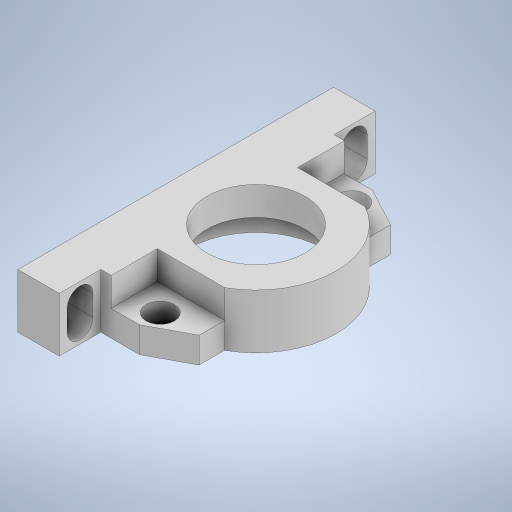
# Autodesk Inventor part: clock_part1
Saved by Autodesk Inventor 2024 (Build 280153000, 153)
## iProperties
Created: 2024-10-24
Part Number: clock_part1
Material: Generic
Document SubType Name: Modeling
Designer: Logan
Density: 1 g/cm^3
Appearance: Default
Author: Logan
Autodesk Inventor part; units mm, degrees
ref_plane "YZ Plane" through (0, 0, 0) normal (1, 0, 0) x (0, 1, 0)
ref_plane "XZ Plane" through (0, 0, 0) normal (0, 1, 0) x (-1, 0, 0)
ref_plane "XY Plane" through (0, 0, 0) normal (0, 0, 1) x (1, 0, 0)
sketch "Sketch1" plane through (0, 0, 0) normal (0, 1, 0) x (-1, 0, 0)
  circle A0 centre (0, 0) radius 13
  circle A1 centre (0, 0) radius 15.5
  circle A2 centre (0, 18.5) radius 2.75
  circle A3 centre (0, -18.5) radius 2.75
  line L0 (0, 18.5) -> (0, -18.5)
  line L1 (7.5, 22.5) -> (-7.5, 22.5)
  line L2 (-7.5, 22.5) -> (-7.5, 13)
  line L3 (-7.5, 13) -> (7.5, 13)
  line L4 (7.5, 13) -> (7.5, 22.5)
  line L5 (0, 22.5) -> (7.5, 18.5)
  line L6 (7.5, 18.5) -> (7.5, 13.5647)
  line L7 (0, 22.5) -> (-7.5, 18.5)
  line L8 (-7.5, 18.5) -> (-7.5, 13.5647)
  line L9 (13, 0) -> (-13, 0) construction
  circle A4 centre (0, -18.5) radius 2.75
  line L10 (7.5, -22.5) -> (-7.5, -22.5)
  line L11 (-7.5, -22.5) -> (-7.5, -13)
  line L12 (7.5, -13) -> (7.5, -22.5)
  line L13 (0, -22.5) -> (7.5, -18.5)
  line L14 (0, -22.5) -> (-7.5, -18.5)
  point P0 (-7.5, -13.5647)
  point P1 (7.5, -13.5647)
  dimension "d0" = 26
  dimension "d1" = 2.5
  dimension "d2" = 5.5
  dimension "d3" = 5.5
  dimension "d4" = 37
  dimension "d5" = 15
  dimension "d6" = 4
  constraints: 30 end point, 7 symmetric about line, 6 point on line, 5 centre point, 4 coincident, 4 point on circle, 2 horizontal, 2 midpoint, 2 parallel, 2 vertical alignment, 1 perpendicular, 1 tangent, 1 vertical, 1 other
  measures "d0" diameter of A0
  measures "d1" radial gap between concentric circles of A0 A1
  measures "d2" diameter of A2
  measures "d3" diameter of A3
  measures "d4" distance of L0.end L0.start
  measures "d5" distance of L3.end L2.end
  measures "d6" distance of L5.start L0.start
extrude "Extrusion1" add sketch "Sketch1" along normal blind 5 contours A0 L3 L4 A1 L0 | L3 L2 A1 L0 | A0 L0 A1 L2 L3 | L0 A1 L4 L3 | A1 L2 L7 L5 L4 | A1 L12 L13 L14 L11
sketch "Sketch2" plane through (0, 0, 0) normal (0, -1, 0) x (1, 0, 0)
  line L0 (7.5, -18.5) -> (0, -22.5) projected
  line L1 (0, -22.5) -> (-15.5, -22.5)
  line L2 (-15.5, -22.5) -> (-15.5, 22.5)
  line L3 (-15.5, 22.5) -> (0, 22.5)
  arc A0 (-7.5, 13.5647) -> (-7.5, -13.5647) centre (0, 0) ccw projected
  line L4 (-7.5, 13.5647) -> (-7.5, 18.5) projected
  line L5 (0, 22.5) -> (-7.5, 18.5)
  line L6 (-7.5, 18.5) -> (-7.5, 13.5647)
  arc A1 (-7.5, 13.5647) -> (-15.5, 0) centre (0, 0) ccw
  line L7 (0, -22.5) -> (-7.5, -18.5) projected
  line L8 (0, -22.5) -> (-7.5, -18.5)
  line L9 (-7.5, -18.5) -> (-7.5, -13.5647)
  line L10 (-7.5, -18.5) -> (-7.5, -13.5647) projected
  arc A2 (-7.5, 13.5647) -> (-7.5, -13.5647) centre (0, 0) ccw
  point P0 (-15.5, 0)
  constraints: 14 end point, 5 point on circle, 3 equal length, 2 centre point, 2 coincident, 1 concentric, 1 horizontal, 1 parallel, 1 point on line, 1 tangent, 1 vertical
extrude "Extrusion2" add sketch "Sketch2" against normal up to surface (5 mm away)
sketch "Sketch4" plane through (0, 5, 0) normal (0, 1, 0) x (1, 0, 0)
  arc A0 (7.5, -13.5647) -> (7.5, 13.5647) centre (0, 0) ccw projected
  arc A1 (7.5, -13.5647) -> (7.5, 13.5647) centre (0, 0) ccw
  line L0 (7.5, 13.5647) -> (7.5, 18.5) projected
  line L1 (7.5, 13.5647) -> (-5.5, 13.5647)
  line L2 (-5.5, 13.5647) -> (-5.5, 22.5742)
  line L3 (-5.5, 22.5742) -> (-15.5, 22.5742)
  line L4 (-15.5, -22.5) -> (-15.5, 22.5) projected
  line L5 (-15.5, 22.5742) -> (-15.5, -22.5)
  line L6 (0, -22.5) -> (-15.5, -22.5) projected
  line L7 (-15.5, -22.5) -> (-5.5, -22.5)
  line L8 (-5.5, -22.5) -> (-5.5, -13.5647)
  line L9 (-5.5, -13.5647) -> (7.5, -13.5647)
  line L10 (7.5, -18.5) -> (7.5, -13.5647) projected
  circle A2 centre (0, 0) radius 9.5
  point P0 (-15.5, -30.5)
  point P1 (-15.5, 30.5)
  point P2 (-10, -22.5)
  point P3 (-15.5, -22.5)
  point P4 (-5.5, -22.5)
  point P5 (-5.5, -22.5)
  dimension "d21" = 13
  dimension "d22" = 13
  dimension "d23" = 19
  constraints: 14 end point, 5 perpendicular, 2 centre point, 2 horizontal, 2 point on circle, 1 coincident, 1 point on line
  measures "d21" distance between parallel lines of L2 L0
  measures "d22" distance between parallel lines of L8 L10
  measures "d23" diameter of A2
extrude "Extrusion4" add sketch "Sketch4" along normal blind 5.5
sketch "Sketch5" plane through (-15.5, 0, -22.5) normal (-1, 0, 0) x (0, 0, 1)
  line L0 (45, 0) -> (45, 5) projected
  line L1 (45, 0) -> (53, 0)
  line L2 (53, 0) -> (53, 10.5)
  line L3 (53, 10.5) -> (45, 10.5)
  line L4 (45, 10.5) -> (45, 0)
  line L5 (4, 0) -> (0, 0) projected
  line L6 (0, 0) -> (-8, 0)
  line L7 (-8, 0) -> (-8, 10.5)
  line L8 (-8, 10.5) -> (0, 10.5)
  line L9 (0, 10.5) -> (0, 0)
  line L10 (-0.0742, 10.5) -> (45, 10.5) projected
  line L11 (-4, 3.25) -> (-4, 7.25) construction
  line L12 (-1.5, 3.25) -> (-1.5, 7.25)
  line L13 (-6.5, 7.25) -> (-6.5, 3.25)
  arc A0 (-6.5, 3.25) -> (-1.5, 3.25) centre (-4, 3.25) ccw
  arc A1 (-1.5, 7.25) -> (-6.5, 7.25) centre (-4, 7.25) ccw
  line L14 (49, 3.25) -> (49, 7.25) construction
  line L15 (51.5, 3.25) -> (51.5, 7.25)
  line L16 (46.5, 7.25) -> (46.5, 3.25)
  arc A2 (46.5, 3.25) -> (51.5, 3.25) centre (49, 3.25) ccw
  arc A3 (51.5, 7.25) -> (46.5, 7.25) centre (49, 7.25) ccw
  point P0 (22.5, 0)
  point P1 (49, 10.5)
  point P2 (0, 5.25)
  point P3 (-4, 5.25)
  point P4 (-4, 0)
  point P5 (-6.5, 5.25)
  point P6 (49, 5.25)
  point P7 (46.5, 5.25)
  point P8 (45, 5.25)
  dimension "d26" = 8
  dimension "d27" = 8
  dimension "d28" = 0
  dimension "d29" = 4
  dimension "d30" = 5
  dimension "d31" = 4
  dimension "d32" = 5
  constraints: 32 end point, 8 midpoint, 8 point on circle, 8 tangent, 6 parallel, 4 centre point, 3 horizontal alignment, 2 horizontal, 2 perpendicular, 2 vertical, 2 vertical alignment
  measures "d26" distance of L3.end L2.end
  measures "d27" distance from line of point (0, 5.25) L7
  measures "d28" distance between parallel lines of L10 L8
  measures "d29" distance of L11.start L11.end
  measures "d30" distance from line of point (-6.5, 5.25) L12
  measures "d31" distance of L14.start L14.end
  measures "d32" distance from line of point (46.5, 5.25) L15
extrude "Extrusion5" add sketch "Sketch5" against normal blind 8
body "Solid1"
